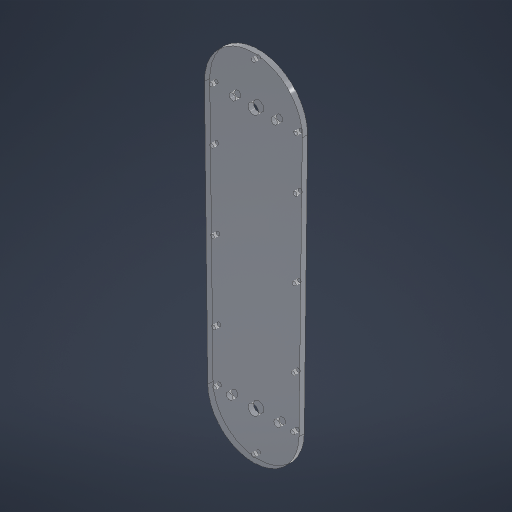
# Autodesk Inventor part: 4ELO
Saved by Autodesk Inventor 2025.2 (Build 292293000, 293)
## iProperties
Created: 2025-05-02
Part Number: 4ELO
Material: Generic
Document SubType Name: Modeling
Designer: Nelson
Density: 1 g/cm^3
Appearance: Polycarbonate - Clear
Author: Nelson
Autodesk Inventor part; units mm, degrees
ref_plane "YZ Plane" through (0, 0, 0) normal (1, 0, 0) x (0, 1, 0)
ref_plane "XZ Plane" through (0, 0, 0) normal (0, 1, 0) x (-1, 0, 0)
ref_plane "XY Plane" through (0, 0, 0) normal (0, 0, 1) x (1, 0, 0)
sketch "Sketch1" plane through (0, 0, 0) normal (0, 0, 1) x (1, 0, 0)
  arc A0 (37.4971, -0.4687) -> (-37.4971, -0.4688) centre (0, 0) ccw
  line L0 (0, 0) -> (0, -200) construction
  arc A1 (-35, -200) -> (35, -200) centre (0, -200) ccw
  circle A2 centre (0, -200) radius 4
  circle A3 centre (0, 0) radius 4
  line L1 (0, -200) -> (18.25, -200) construction
  circle A4 centre (18.25, -200) radius 2.5
  circle A5 centre (0, -200) radius 21 construction
  line L2 (0, -235) -> (0, -230) construction
  circle A6 centre (0, -230) radius 1.5
  line L3 (37.4971, -0.4687) -> (34.9973, -200.4375)
  line L4 (-37.4971, -0.4688) -> (-34.9973, -200.4375)
  line L5 (36.2472, -100.4531) -> (31.2476, -100.3906) construction
  line L6 (30.4976, -160.3859) -> (31.9976, -40.3953) construction
  circle A7 centre (31.9976, -40.3953) radius 1.5
  circle A8 centre (31.2476, -100.3906) radius 1.5
  circle A9 centre (30.4976, -160.3859) radius 1.5
  line L7 (37.5, 0) -> (32.5, 0) construction
  line L8 (0, 37.5) -> (0, 32.5) construction
  circle A10 centre (0, 32.5) radius 1.5
  circle A11 centre (32.5, 0) radius 1.5
  line L9 (35, -200) -> (30, -200) construction
  circle A12 centre (30, -200) radius 1.5
  circle A13 centre (-31.9976, -40.3953) radius 1.5
  circle A14 centre (-31.2476, -100.3906) radius 1.5
  circle A15 centre (-30.4976, -160.3859) radius 1.5
  circle A16 centre (-32.5, 0) radius 1.5
  line L10 (-35, -200) -> (-30, -200) construction
  circle A17 centre (-30, -200) radius 1.5
  line L11 (0, 0) -> (16, 0) construction
  circle A18 centre (16, 0) radius 2.5
  line L12 (0, -200) -> (-18.25, -200) construction
  circle A19 centre (-18.25, -200) radius 2.5
  line L13 (0, 0) -> (-16, 0) construction
  circle A20 centre (-16, 0) radius 2.5
  line L14 (0, -200) -> (0, -60.58) construction
  dimension "D_Junta2" = 75
  dimension "L_Elo" = 200
  dimension "D_Junta3" = 70
  dimension "Veio" = 8
  dimension "d4" = 8
  dimension "d5" = 18.25
  dimension "d6" = 5
  dimension "D_P" = 42
  dimension "LF" = 5
  dimension "D_Sup" = 3
  dimension "d10" = 5
  dimension "d12" = 120
  dimension "d13" = 3
  dimension "d14" = 3
  dimension "d15" = 3
  dimension "d16" = 5
  dimension "d17" = 5
  dimension "d18" = 3
  dimension "d19" = 3
  dimension "d20" = 5
  dimension "d21" = 3
  dimension "d22" = 16
  dimension "d23" = 5
  dimension "d26" = 139.42
  constraints: 30 end point, 21 centre point, 21 coincident, 16 symmetric about line, 9 point on circle, 4 horizontal, 4 line through centre, 4 tangent, 3 vertical, 2 midpoint, 1 parallel, 1 perpendicular, 1 point on line, 7 other
  measures "D_Junta2" diameter of A0
  measures "L_Elo" distance of L0.start L0.end
  measures "D_Junta3" diameter of A1
  measures "Veio" diameter of A2
  measures "d4" diameter of A3
  measures "d5" distance of L0.end L1.end
  measures "d6" diameter of A4
  measures "D_P" diameter of A5
  measures "LF" distance of L2.start L2.end
  measures "D_Sup" diameter of A6
  measures "d10" distance of L5.start L5.end
  measures "d12" distance of L6.start L6.end
  measures "d13" diameter of A7
  measures "d14" diameter of A8
  measures "d15" diameter of A9
  measures "d16" distance of L7.start L7.end
  measures "d17" distance of L8.start L8.end
  measures "d18" diameter of A10
  measures "d19" diameter of A11
  measures "d20" distance of L9.start L9.end
  measures "d21" diameter of A12
  measures "d22" distance of L11.start L11.end
  measures "d23" diameter of A18
  measures "d26" distance of L12.start L14.end
extrude "Extrusion1" add sketch "Sketch1" along normal blind 4
sketch "Sketch2" plane through (0, 0, 4) normal (0, 0, 1) x (1, 0, 0)
  line L0 (0, 0) -> (0, 36)
  line L1 (-0.005, 35.995) -> (0.005, 35.995)
  line L2 (0.005, 35.995) -> (0.005, 36.005)
  line L3 (0.005, 36.005) -> (-0.005, 36.005)
  line L4 (-0.005, 36.005) -> (-0.005, 35.995)
  line L5 (-0.005, 35.995) -> (0.005, 36.005) construction
  line L6 (0.005, 35.995) -> (-0.005, 36.005) construction
  dimension "d28" = 36
  dimension "d29" = 0.01
  dimension "d30" = 0.01
  constraints: 14 end point, 2 midpoint, 2 parallel, 1 horizontal, 1 perpendicular, 1 vertical
  measures "d28" distance of L0.start L0.end
  measures "d29" distance of L3.end L2.end
  measures "d30" distance of L1.end L2.end
extrude "Extrusion2" add sketch "Sketch2" along normal blind 0.01
equation "\"d4\" = Veio"
equation "\"d10\" = LF"
equation "\"d13\" = D_Sup"
equation "\"d14\" = D_Sup"
equation "\"d15\" = D_Sup"
equation "\"d16\" = LF"
equation "\"d17\" = LF"
equation "\"d18\" = D_Sup"
equation "\"d19\" = D_Sup"
equation "\"d20\" = LF"
equation "\"d21\" = D_Sup"
body "Solid1"
